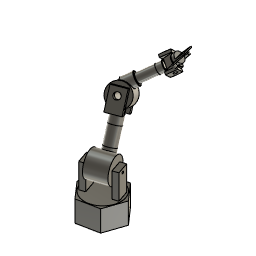
Robotic ARM v11 (Autodesk Fusion 360 design; units mm, degrees)
Autodesk Fusion 360 part; units mm, degrees
(part 1 of 2)
sketch "Sketch7" plane through (0, 0, 0) normal (0, 0, 1) x (1, 0, 0)
  line L0 (526.8037, -602.0614) -> (784.8023, 155.1947)
  line L1 (784.8023, 155.1947) -> (257.9986, 757.2561)
  line L2 (257.9986, 757.2561) -> (-526.8037, 602.0614)
  line L3 (-526.8037, 602.0614) -> (-784.8023, -155.1947)
  line L4 (-784.8023, -155.1947) -> (-257.9986, -757.2561)
  line L5 (-257.9986, -757.2561) -> (526.8037, -602.0614)
  circle A0 centre (0, 0) radius 667.5
  dimension "d16" = 800
  dimension "d17" = 1335
  constraint coincident A0.centre origin
  measures "d16" distance of L0.start A0.centre
  measures "d17" diameter of A0
extrude "Extrude5" add sketch "Sketch7" along normal blind 770 makes body 1
sketch "Sketch8" plane through (0, 0, 0) normal (0, 0, 1) x (1, 0, 0)
  circle A0 centre (0, 0) radius 630
  dimension "d20" = 1260
  constraint coincident A0.centre origin
  measures "d20" diameter of A0
extrude "Extrude6" add sketch "Sketch8" along normal blind 65 from surface at 770 separate body makes body 2
sketch "Sketch9" plane through (0, 0, 835) normal (0, 0, 1) x (-1, 0, 0)
  circle A0 centre (0, 0) radius 630
  line L0 (0, -630) -> (0, 630)
  line L1 (0, -630) -> (0, -480)
  line L2 (0, 630) -> (0, 480)
  line L3 (225, -380) -> (-225, -380)
  line L4 (-225, -380) -> (-225, -580)
  line L5 (-225, -580) -> (225, -580)
  line L6 (225, -580) -> (225, -380)
  line L7 (225, -380) -> (-225, -580) construction
  line L8 (-225, -380) -> (225, -580) construction
  line L9 (-225, 380) -> (225, 380)
  line L10 (225, 380) -> (225, 580)
  line L11 (225, 580) -> (-225, 580)
  line L12 (-225, 580) -> (-225, 380)
  line L13 (-225, 380) -> (225, 580) construction
  line L14 (225, 380) -> (-225, 580) construction
  point P0 (0, -480)
  point P1 (0, 480)
  dimension "d24" = 150
  dimension "d25" = 150
  dimension "d26" = 450
  dimension "d27" = 200
  dimension "d28" = 450
  dimension "d29" = 200
  constraint coincident A0 L0.start
  constraint coincident A0 L0.end
  constraint vertical L0
  constraint parallel L0 L1
  constraint parallel L0 L2
  constraint horizontal L3
  constraint perpendicular L3 L4
  constraint parallel L3 L5
  constraint parallel L4 L6
  constraint coincident L7 P0
  constraint coincident L8 P0
  constraint coincident P0 L1.end
  constraint horizontal L9
  constraint perpendicular L9 L10
  constraint parallel L9 L11
  constraint parallel L10 L12
  constraint coincident L13 P1
  constraint coincident L14 P1
  constraint coincident P1 L2.end
  measures "d24" distance of L0.start P0
  measures "d25" distance of L0.end P1
  measures "d26" distance of L4.end L5.end
  measures "d27" distance of L3.end L4.end
  measures "d28" distance of L10.end L11.end
  measures "d29" distance of L9.end L10.end
extrude "Extrude7" add sketch "Sketch9" along normal blind 900 contours L0 L2 L9 L10 L11 | L0 L2 L9 L11 L12 | L0 L1 L3 L4 L5 | L0 L1 L3 L5 L6 bodies 2
sketch "Sketch10" plane through (0, 580, 0) normal (0, 1, 0) x (-1, 0, 0)
  line L0 (-225, 835) -> (225, 835)
  line L1 (225, 835) -> (225, 1735)
  line L2 (225, 1735) -> (-225, 1735)
  line L3 (-225, 1735) -> (-225, 835)
  line L4 (0, 835) -> (0, 1602)
  circle A0 centre (0, 1602) radius 42
  circle A1 centre (0, 1602) radius 440
  dimension "d32" = 767
  dimension "d33" = 84
  dimension "d34" = 880
  constraint midpoint L0 L4.start
  constraint perpendicular L0 L4
  constraint coincident L4.end A0.centre
  constraint concentric A0 A1
  measures "d32" distance of L4.start L4.end
  measures "d33" diameter of A0
  measures "d34" diameter of A1
extrude "Extrude8" cut sketch "Sketch10" against normal blind 1300 contours A0 bodies 2
sketch "Sketch11" plane through (0, 580, 0) normal (0, 1, 0) x (-1, 0, 0)
  circle A0 centre (0, 1602) radius 42
  line L0 (-225, 835) -> (225, 835)
  line L1 (225, 835) -> (225, 1735)
  line L2 (225, 1735) -> (-225, 1735)
  line L3 (-225, 1735) -> (-225, 835)
  circle A1 centre (0, 1602) radius 440
  dimension "d37" = 880
  constraint concentric A0 A1
  measures "d37" diameter of A1
extrude "Extrude9" add sketch "Sketch11" against normal blind 715 from surface at -225 separate body contours L1 L2 L3 A1 | L1 L2 L3 A1 makes body 3
sketch "Sketch12" plane through (0, 0, 835) normal (0, 0, 1) x (-1, 0, 0)
  line L0 (225, -580) -> (-225, -580)
  line L1 (-225, -580) -> (-225, -380)
  line L2 (-225, -380) -> (225, -380)
  line L3 (225, -380) -> (225, -580)
  line L4 (-225, 580) -> (225, 580)
  line L5 (225, 580) -> (225, 380)
  line L6 (225, 380) -> (-225, 380)
  line L7 (-225, 380) -> (-225, 580)
  circle A0 centre (0, 0) radius 630
  circle A1 centre (200, 0) radius 205
  dimension "d44" = 410
  measures "d44" diameter of A1
sketch "Sketch13" plane through (0, 0, 770) normal (0, 0, -1) x (1, 0, 0)
  circle A0 centre (0, 0) radius 630
  circle A1 centre (0, 0) radius 667
  dimension "d41" = 1334
  constraint concentric A0 A1
  measures "d41" diameter of A1
extrude "Extrude10" add sketch "Sketch13" against normal blind 65 bodies 2
sketch "Sketch14" plane through (0, 0, 0) normal (0, 1, 0) x (1, 0, 0)
sketch "Sketch15" plane through (0, 0, 835) normal (0, 0, 1) x (-1, 0, 0)
copy_body "Body->Comp2" bodies 3 removing the originals makes body 4 in component "old_component (1)"
copy_body "Body->Comp3" bodies 2 removing the originals makes body 5 in component "old_component (2)"
copy_body "Body->Comp4" bodies 1 removing the originals makes body 6 in component "old_component"
extrude "Extrude1" add 1 faces at (176.6231, 355, 1351.5163) along direction (0, 1, 0) blind 20 on bodies 4 bodies 4 in component "old_component (1)"
sketch "Sketch16" plane through (0, 0, 770) normal (0, 0, 1) x (-1, 0, 0)
  circle A0 centre (0, 0) radius 667
  line L0 (225, -580) -> (-225, -580)
  line L1 (-225, -580) -> (-225, -380)
  line L2 (-225, -380) -> (225, -380)
  line L3 (225, -380) -> (225, -580)
  line L4 (-225, 580) -> (225, 580)
  line L5 (225, 580) -> (225, 380)
  line L6 (225, 380) -> (-225, 380)
  line L7 (-225, 380) -> (-225, 580)
  circle A1 centre (200, 0) radius 205
  dimension "d60" = 410
  measures "d60" diameter of A1
extrude "Extrude2" add sketch "Sketch16" along normal blind 400 and the other way blind 0 from surface at 900 contours A1 sketch seen with x (1, 0, 0) y (0, 1, 0) z (0, 0, 1) at (0, 7.5, 65) bodies 4 in component "old_component (1)"
sketch "Sketch17" plane through (0, 0, 1880.3087) normal (0, 0, 1) x (-1, 0, 0)
  circle A0 centre (137.9029, 21.8013) radius 205
  circle A1 centre (137.9029, 21.8013) radius 204
  dimension "d66" = 408
  constraint concentric A0 A1
  measures "d66" diameter of A1
extrude "Extrude3" cut sketch "Sketch17" against normal blind 300 contours A1 sketch seen with x (1, 0, 0) y (0, 1, 0) z (0, 0, 1) at (-62.0971, 29.3013, 254.6913) bodies 4 in component "old_component (1)"
sketch "Sketch18" plane through (0, 0, 1633.8201) normal (0, 0, 1) x (-1, 0, 0)
  circle A0 centre (38.5203, 22.1078) radius 204
extrude "Extrude4" add sketch "Sketch18" along normal blind 1200 sketch seen with x (1, 0, 0) y (0, 1, 0) z (0, 0, 1) at (-161.4797, 29.6078, 201.1799) bodies 4 in component "old_component (1)"
sketch "Sketch19" plane through (0, 0, 2833.8201) normal (0, 0, 1) x (-1, 0, 0)
  circle A0 centre (38.5203, 22.1078) radius 204
  circle A1 centre (38.5203, 22.1078) radius 205
  dimension "d71" = 410
  constraint concentric A0 A1
  measures "d71" diameter of A1
extrude "Extrude12" add sketch "Sketch19" against normal blind 300 separate body contours A0 makes body 7
sketch "Sketch20" plane through (0, 0, 2833.8201) normal (0, 0, 1) x (-1, 0, 0)
  circle A0 centre (38.5203, 22.1078) radius 204
  line L0 (-165.4797, 22.1078) -> (-415.4797, 22.1078)
  line L1 (-415.4797, 22.1078) -> (-415.4797, -227.8922)
  line L2 (-415.4797, 22.1078) -> (-415.4797, 272.1078)
  line L3 (242.5203, 22.1078) -> (492.5203, 22.1078)
  line L4 (492.5203, 22.1078) -> (492.5203, 272.1078)
  line L5 (492.5203, 22.1078) -> (492.5203, -227.8922)
  line L6 (38.5203, 22.1078) -> (-261.4797, 22.1078)
  line L7 (38.5203, 22.1078) -> (338.5203, 22.1078)
  line L8 (338.5203, 22.1078) -> (338.5203, -227.8922)
  line L9 (338.5203, -227.8922) -> (492.5203, -227.8922)
  line L10 (492.5203, 272.1078) -> (338.5203, 272.1078)
  line L11 (338.5203, 272.1078) -> (338.5203, 22.1078)
  line L12 (-261.4797, 22.1078) -> (-261.4797, 272.1078)
  line L13 (-261.4797, 272.1078) -> (-415.4797, 272.1078)
  line L14 (-261.4797, 22.1078) -> (-261.4797, -227.8922)
  line L15 (-261.4797, -227.8922) -> (-415.4797, -227.8922)
  line L16 (-261.4797, 22.1078) -> (-261.4797, 147.1078)
  line L17 (338.5203, 147.1078) -> (338.5203, -102.8922)
  line L18 (-261.4797, -102.8922) -> (338.5203, -102.8922)
  line L19 (338.5203, 147.1078) -> (-261.4797, 147.1078)
  point P0 (-165.4797, 22.1078)
  dimension "d74" = 250
  dimension "d76" = 250
  dimension "d77" = 250
  dimension "d80" = 250
  dimension "d81" = 250
  dimension "d82" = 250
  dimension "d83" = 300
  dimension "d84" = 300
  constraint coincident P0 L0.start
  constraint horizontal L0
  constraint perpendicular L0 L1
  constraint perpendicular L0 L2
  constraint coincident A0 L3.start
  constraint parallel L0 L3
  constraint perpendicular L3 L4
  constraint perpendicular L3 L5
  constraint coincident A0.centre L6.start
  constraint coincident L0 L6.end
  constraint parallel L3 L7
  constraint perpendicular L7 L8
  constraint perpendicular L5 L9
  constraint perpendicular L8 L10
  constraint perpendicular L7 L11
  constraint perpendicular L6 L12
  constraint perpendicular L2 L13
  constraint perpendicular L0 L14
  constraint perpendicular L1 L15
  constraint midpoint L12 L16.end
  constraint midpoint L11 L17.start
  constraint midpoint L8 L17.end
  constraint midpoint L14 L18.start
  constraint perpendicular L8 L18
  measures "d74" distance of P0 L0.end
  measures "d76" distance of L0.end L1.end
  measures "d77" distance of L0.end L2.end
  measures "d80" distance of L3.start L3.end
  measures "d81" distance of L3.end L4.end
  measures "d82" distance of L3.end L5.end
  measures "d83" distance of A0.centre L6.end
  measures "d84" distance of A0.centre L7.end
extrude "Extrude13" add sketch "Sketch20" along normal blind 750 contours A0 L6 L7 L19 | A0 L3 L7 L8 L17 L18 | A0 L3 L7 L11 L17 L19 | A0 L6 L7 L18 | L3 L4 L10 L11 L17 | L3 L5 L8 L9 L17 | A0 L0 L6 L12 L16 L19 | A0 L0 L6 L14 L18 | L0 L2 L12 L13 L16 | L0 L1 L14 L15 bodies 7
sketch "Sketch21" plane through (0, 0, 3583.8201) normal (0, 0, 1) x (-1, 0, 0)
  line L0 (492.5203, -227.8922) -> (492.5203, 272.1078)
  line L1 (492.5203, 272.1078) -> (338.5203, 272.1078)
  line L2 (338.5203, 272.1078) -> (338.5203, 147.1078)
  line L3 (338.5203, 147.1078) -> (-261.4797, 147.1078)
  line L4 (-261.4797, 147.1078) -> (-261.4797, 272.1078)
  line L5 (-261.4797, 272.1078) -> (-415.4797, 272.1078)
  line L6 (-415.4797, 272.1078) -> (-415.4797, -227.8922)
  line L7 (-415.4797, -227.8922) -> (-261.4797, -227.8922)
  line L8 (-261.4797, -227.8922) -> (-261.4797, -102.8922)
  line L9 (-261.4797, -102.8922) -> (338.5203, -102.8922)
  line L10 (338.5203, -102.8922) -> (338.5203, -227.8922)
  line L11 (338.5203, -227.8922) -> (492.5203, -227.8922)
  line L12 (-261.4797, 147.1078) -> (-261.4797, -102.8922)
  line L13 (338.5203, -102.8922) -> (338.5203, 147.1078)
  line L14 (-261.4797, 147.1078) -> (-261.4797, -102.8922)
  line L15 (338.5203, -102.8922) -> (-261.4797, -102.8922)
  line L16 (-261.4797, 147.1078) -> (338.5203, 147.1078)
  constraint coincident L3.end L4.start
  constraint coincident L8.end L9.start
  constraint coincident L9.end L10.start
  constraint coincident L2.end L3.start
extrude "Extrude14" cut sketch "Sketch21" against normal blind 600 contours L3 L9 L12 L13 L14 L15 L16 bodies 7
sketch "Sketch22" plane through (-492.5203, 0, 0) normal (-1, 0, 0) x (0, -1, 0)
  line L0 (-227.8922, 2833.8201) -> (272.1078, 2833.8201)
  line L1 (272.1078, 2833.8201) -> (272.1078, 3583.8201)
  line L2 (272.1078, 3583.8201) -> (-227.8922, 3583.8201)
  line L3 (-227.8922, 3583.8201) -> (-227.8922, 2833.8201)
  line L4 (22.1078, 2833.8201) -> (22.1078, 3333.8201)
  circle A0 centre (22.1078, 3333.8201) radius 112
  dimension "d89" = 500
  dimension "d90" = 224
  constraint midpoint L0 L4.start
  constraint perpendicular L0 L4
  constraint coincident L4.end A0.centre
  measures "d89" distance of L4.start L4.end
  measures "d90" diameter of A0
extrude "Extrude15" cut sketch "Sketch22" against normal blind 2400 contours A0 bodies 7
sketch "Sketch23" plane through (415.4797, 0, 0) normal (1, 0, 0) x (0, 1, 0)
  circle A0 centre (-22.1078, 3333.8201) radius 112
  line L0 (-272.1078, 2833.8201) -> (227.8922, 2833.8201)
  line L1 (227.8922, 2833.8201) -> (227.8922, 3583.8201)
  line L2 (227.8922, 3583.8201) -> (-272.1078, 3583.8201)
  line L3 (-272.1078, 3583.8201) -> (-272.1078, 2833.8201)
  circle A1 centre (-22.1078, 3333.8201) radius 390
  dimension "d97" = 780
  constraint concentric A0 A1
  measures "d97" diameter of A1
extrude "Extrude16" add sketch "Sketch23" against normal blind 600 from surface at -150 separate body contours L1 L2 L3 A1 | L1 L2 L3 A1 makes body 8
sketch "Sketch24" plane through (0, 0, 3583.8201) normal (0, 0, 1) x (-1, 0, 0)
  line L0 (338.5203, 272.1078) -> (338.5203, -227.8922)
  line L1 (338.5203, -227.8922) -> (492.5203, -227.8922)
  line L2 (492.5203, -227.8922) -> (492.5203, 272.1078)
  line L3 (492.5203, 272.1078) -> (338.5203, 272.1078)
  circle A0 centre (33.0014, 228.1503) radius 222.5
  dimension "d101" = 445
  measures "d101" diameter of A0
extrude "Extrude17" add sketch "Sketch24" along normal blind 200 and the other way blind 100 contours A0 bodies 8
extrude "Extrude18" add 1 faces at (-79.2435, -170.1644, 3783.8201) along direction (0, 0, 1) blind 0 and the other way blind 300 separate body on bodies 8 makes body 9
extrude "Extrude19" add 1 faces at (-79.2435, -170.1644, 3783.8201) along direction (0, 0, 1) blind 100 on bodies 8 bodies 8 9
sketch "Sketch25" plane through (0, 0, 3883.8201) normal (0, 0, 1) x (-1, 0, 0)
  circle A0 centre (33.0014, 228.1503) radius 222.5
  circle A1 centre (33.0014, 228.1503) radius 200
  dimension "d112" = 400
  constraint concentric A0 A1
  measures "d112" diameter of A1
extrude "Extrude20" add sketch "Sketch25" along normal blind 15 contours A1 bodies 8
sketch "Sketch26" plane through (0, 0, 3898.8201) normal (0, 0, 1) x (-1, 0, 0)
  circle A0 centre (33.0014, 228.1503) radius 200
  circle A1 centre (33.0014, 228.1503) radius 155
  dimension "d115" = 310
  constraint concentric A0 A1
  measures "d115" diameter of A1
extrude "Extrude21" add sketch "Sketch26" along normal blind 900 separate body contours A1 makes body 10
sketch "Sketch27" plane through (0, 0, 4798.8201) normal (0, 0, 1) x (-1, 0, 0)
  circle A0 centre (33.0014, 228.1503) radius 155
  circle A1 centre (33.0014, 228.1503) radius 162.5
  dimension "d118" = 325
  constraint concentric A0 A1
  measures "d118" diameter of A1
extrude "Extrude22" add sketch "Sketch27" along normal blind 200 separate body makes body 11
sketch "Sketch28" plane through (0, 0, 4998.8201) normal (0, 0, 1) x (-1, 0, 0)
  circle A0 centre (33.0014, 228.1503) radius 155
  circle A1 centre (33.0014, 228.1503) radius 162.5
  circle A2 centre (33.0014, 228.1503) radius 155
  constraint concentric A0 A2
extrude "Extrude23" add sketch "Sketch28" against normal blind 1 contours A0 A2 bodies 11
sketch "Sketch29" plane through (0, 0, 4998.8201) normal (0, 0, 1) x (-1, 0, 0)
  circle A0 centre (33.0014, 228.1503) radius 162.5
  line L0 (33.0014, 228.1503) -> (-171.9986, 228.1503)
  line L1 (-171.9986, 228.1503) -> (238.0014, 228.1503)
  line L2 (-129.4986, 228.1503) -> (-126.7294, 258.0222)
  line L3 (-129.4986, 228.1503) -> (-126.7294, 198.2784)
  line L4 (-126.7294, 198.2784) -> (-171.9986, 198.2784)
  line L5 (-126.7294, 258.0222) -> (-171.9986, 258.0222)
  line L6 (-171.9986, 258.0222) -> (-171.9986, 228.1503)
  line L7 (-171.9986, 198.2784) -> (-171.9986, 228.1503)
  line L8 (195.5014, 228.1503) -> (192.7321, 258.0222)
  line L9 (195.5014, 228.1503) -> (192.7203, 198.2155)
  line L10 (238.0014, 228.1503) -> (238.0014, 198.2155)
  line L11 (238.0014, 198.2155) -> (192.7203, 198.2155)
  line L12 (238.0014, 258.0222) -> (192.7321, 258.0222)
  line L13 (238.0014, 258.0222) -> (238.0014, 228.1503)
  point P0 (-129.4986, 228.1503)
  dimension "d123" = 205
  dimension "d124" = 410
  dimension "d126" = 30
  dimension "d127" = 30
  dimension "d128" = 30
  constraint coincident A0.centre L0.start
  constraint horizontal L0
  constraint parallel L0 L1
  constraint coincident P0 L2.start
  constraint coincident A0 L2.end
  constraint coincident A0 L3.end
  constraint parallel L1 L4
  constraint parallel L0 L5
  constraint perpendicular L5 L6
  constraint perpendicular L1 L7
  constraint coincident L1 L8.start
  constraint coincident A0 L8.start
  constraint coincident A0 L8.end
  constraint coincident A0 L9.end
  constraint perpendicular L1 L10
  constraint perpendicular L10 L11
  constraint parallel L1 L12
  constraint perpendicular L1 L13
  measures "d123" distance of A0.centre L0.end
  measures "d124" distance of L0.end L1.end
  measures "d126" distance of P0 L2.end
  measures "d127" distance of P0 L3.end
  measures "d128" distance of L8.start L8.end
extrude "Extrude24" add sketch "Sketch29" along normal blind 10 contours A0 L1 L10 L11 | A0 L1 L12 L13 | A0 L0 L1 L5 L6 | A0 L0 L1 L4 L7 bodies 11
sketch "Sketch30" plane through (0, 0, 5008.8201) normal (0, 0, 1) x (-1, 0, 0)
  line L0 (-126.7294, 258.0222) -> (-171.9986, 258.0222)
  line L1 (-171.9986, 258.0222) -> (-171.9986, 198.2784)
  line L2 (-171.9986, 198.2784) -> (-126.7294, 198.2784)
  arc A0 (-126.7294, 258.0222) -> (-126.7294, 198.2784) centre (33.0014, 228.1503) ccw
  line L3 (-171.9986, 198.2784) -> (-171.9986, 48.2784)
  line L4 (-171.9986, 258.0222) -> (-171.9986, 408.0222)
  line L5 (-171.9986, 408.0222) -> (-261.9986, 408.0222)
  line L6 (-261.9986, 408.0222) -> (-261.9986, 48.2784)
  line L7 (-261.9986, 48.2784) -> (-171.9986, 48.2784)
  line L8 (-171.9986, 198.2784) -> (-171.9986, 258.0222)
  line L9 (238.0014, 258.0222) -> (238.0014, 408.0222)
  line L10 (238.0014, 198.2155) -> (238.0014, 258.0222)
  line L11 (238.0014, 258.0222) -> (238.0014, 198.2832)
  line L12 (238.0014, 198.2832) -> (238.0014, 48.2832)
  line L13 (238.0014, 48.2832) -> (328.0014, 48.2832)
  line L14 (328.0014, 48.2832) -> (328.0014, 408.0222)
  line L15 (328.0014, 408.0222) -> (238.0014, 408.0222)
  point P0 (238.0014, 258.0222)
  dimension "d131" = 150
  dimension "d132" = 150
  dimension "d133" = 90
  dimension "d134" = 150
  dimension "d135" = 150
  dimension "d136" = 90
  constraint coincident L1.end L2.start
  constraint perpendicular L2 L3
  constraint coincident L0.end L1.start
  constraint perpendicular L0 L4
  constraint perpendicular L4 L5
  constraint perpendicular L0 L6
  constraint perpendicular L3 L7
  constraint coincident P0 L9.start
  constraint vertical L9
  constraint coincident L10 L11.end
  constraint parallel L9 L11
  constraint parallel L11 L12
  constraint perpendicular L12 L13
  constraint perpendicular L13 L14
  constraint perpendicular L9 L15
  measures "d131" distance of L1.end L3.end
  measures "d132" distance of L0.end L4.end
  measures "d133" distance of L4.end L5.end
  measures "d134" distance of P0 L9.end
  measures "d135" distance of L11.end L12.end
  measures "d136" distance of L12.end L13.end
extrude "Extrude25" add sketch "Sketch30" along normal blind -10 and the other way blind -400 contours L1 L3 L4 L5 L6 L7 L8 | L9 L10 L11 L12 L13 L14 L15 bodies 11 10 8 7
sketch "Sketch31" plane through (-328.0014, 0, 0) normal (-1, 0, 0) x (0, -1, 0)
  line L0 (48.2832, 5408.8201) -> (48.2832, 4998.8201)
  line L1 (48.2832, 4998.8201) -> (408.0222, 4998.8201)
  line L2 (408.0222, 4998.8201) -> (408.0222, 5408.8201)
  line L3 (408.0222, 5408.8201) -> (48.2832, 5408.8201)
  line L4 (408.0222, 4998.8201) -> (48.2832, 4998.8201)
  line L5 (228.1527, 4998.8201) -> (228.1527, 5148.8201)
  circle A0 centre (228.1527, 5218.8201) radius 70
  dimension "d141" = 150
  dimension "d142" = 140
  constraint coincident L1.end L2.start
  constraint coincident L0.end L1.start
  constraint midpoint L4 L5.start
  constraint perpendicular L4 L5
  constraint coincident L5.end A0
  measures "d141" distance of L5.start L5.end
  measures "d142" diameter of A0
extrude "Extrude26" cut sketch "Sketch31" against normal blind 1400 contours A0 bodies 11
sketch "Sketch32" plane through (261.9986, 0, 0) normal (1, 0, 0) x (0, 1, 0)
  circle A0 centre (-228.1527, 5218.8201) radius 70
  line L0 (-408.0222, 5408.8201) -> (-408.0222, 4998.8201)
  line L1 (-408.0222, 4998.8201) -> (-48.2784, 4998.8201)
  line L2 (-48.2784, 4998.8201) -> (-48.2784, 5408.8201)
  line L3 (-48.2784, 5408.8201) -> (-408.0222, 5408.8201)
  line L4 (-228.1527, 5218.8201) -> (-228.1527, 5048.8201)
  line L5 (-228.1527, 5218.8201) -> (-228.1527, 5388.8201)
  line L6 (-228.1527, 5388.8201) -> (-398.1527, 5388.8201)
  line L7 (-228.1527, 5388.8201) -> (-58.1527, 5388.8201)
  line L8 (-58.1527, 5388.8201) -> (-58.1527, 5048.8201)
  line L9 (-58.1527, 5048.8201) -> (-228.1527, 5048.8201)
  line L10 (-398.1527, 5388.8201) -> (-398.1527, 5048.8201)
  line L11 (-398.1527, 5048.8201) -> (-228.1527, 5048.8201)
  dimension "d145" = 170
  dimension "d146" = 170
  dimension "d147" = 170
  dimension "d148" = 170
  constraint coincident A0.centre L4.start
  constraint vertical L4
  constraint parallel L4 L5
  constraint perpendicular L5 L6
  constraint perpendicular L5 L7
  constraint perpendicular L7 L8
  constraint perpendicular L4 L9
  constraint perpendicular L6 L10
  constraint perpendicular L4 L11
  measures "d145" distance of A0.centre L4.end
  measures "d146" distance of A0.centre L5.end
  measures "d147" distance of L5.end L6.end
  measures "d148" distance of L5.end L7.end
extrude "Extrude27" add sketch "Sketch32" against normal blind 400 from surface at -95 separate body contours A0 L4 L5 | A0 L4 L5 L7 L8 L9 | A0 L4 L5 | A0 L4 L5 L6 L10 L11 makes body 12
extrude "Extrude28" cut 1 faces at (231.9986, -168.193, 5408.8201) along direction (0, 0, -1) blind 50 on bodies 11 bodies 11
extrude "Extrude29" cut 1 faces at (-298.0014, -288.1092, 5408.8201) along direction (0, 0, -1) blind 50 on bodies 11 bodies 11
sketch "Sketch33" plane through (-233.0014, 0, 0) normal (-1, 0, 0) x (0, -1, 0)
  line L0 (398.1527, 5388.8201) -> (58.1527, 5388.8201)
  line L1 (58.1527, 5388.8201) -> (58.1527, 5048.8201)
  line L2 (58.1527, 5048.8201) -> (398.1527, 5048.8201)
  line L3 (398.1527, 5048.8201) -> (398.1527, 5388.8201)
  circle A0 centre (228.1527, 5218.8201) radius 30
  dimension "d156" = 60
  measures "d156" diameter of A0
extrude "Extrude30" cut sketch "Sketch33" against normal blind 900 contours A0 bodies 12
sketch "Sketch34" plane through (0, 0, 5388.8201) normal (0, 0, 1) x (-1, 0, 0)
  line L0 (-166.9986, 398.1527) -> (-166.9986, 58.1527)
  line L1 (-166.9986, 58.1527) -> (233.0014, 58.1527)
  line L2 (233.0014, 58.1527) -> (233.0014, 398.1527)
  line L3 (233.0014, 398.1527) -> (-166.9986, 398.1527)
  line L4 (-166.9986, 228.1527) -> (233.0014, 228.1527)
  line L5 (33.0014, 228.1527) -> (33.0014, 58.1527)
  circle A0 centre (33.0014, 228.1527) radius 180
  dimension "d159" = 360
  constraint midpoint L0 L4.start
  constraint midpoint L2 L4.end
  constraint midpoint L4 L5.start
  constraint midpoint L1 L5.end
  constraint coincident L5.start A0.centre
  measures "d159" diameter of A0
extrude "Extrude31" add sketch "Sketch34" along normal blind 30 contours L3 A0 | L3 L4 A0 | L1 L4 L5 A0 | L1 A0 | L1 L4 L5 A0 bodies 12
extrude "Extrude32" add 1 faces at (-52.7216, -58.1527, 5162.1535) along direction (0, 1, 0) blind 10 on bodies 12 bodies 12
extrude "Extrude33" add 1 faces at (-52.7216, -398.1527, 5162.1535) along direction (0, -1, 0) blind 10 on bodies 12 bodies 12
sketch "Sketch35" plane through (0, 0, 5418.8201) normal (0, 0, 1) x (-1, 0, 0)
  circle A0 centre (33.0014, 228.1527) radius 180
  circle A1 centre (33.0014, 228.1527) radius 180
  dimension "d166" = 360
  constraint concentric A0 A1
  measures "d166" diameter of A1
extrude "Extrude34" add sketch "Sketch35" along normal blind 90 separate body makes body 13
sketch "Sketch36" plane through (0, 0, 5508.8201) normal (0, 0, 1) x (-1, 0, 0)
  circle A0 centre (33.0014, 228.1527) radius 180
  circle A1 centre (33.0014, 228.1527) radius 180
  dimension "d169" = 360
  constraint concentric A0 A1
  measures "d169" diameter of A1
extrude "Extrude35" add sketch "Sketch36" along normal blind 30 bodies 13
sketch "Sketch37" plane through (0, 0, 5538.8201) normal (0, 0, 1) x (-1, 0, 0)
  circle A0 centre (33.0014, 228.1527) radius 180
  line L0 (33.0014, 228.1527) -> (213.0014, 228.1527)
  line L1 (33.0014, 228.1527) -> (-146.9986, 228.1527)
  line L2 (-146.9986, 228.1527) -> (-146.9986, 188.1527)
  line L3 (213.0014, 228.1527) -> (213.0014, 188.1527)
  line L4 (213.0014, 188.1527) -> (-146.9986, 188.1527)
  dimension "d172" = 180
  dimension "d173" = 40
  dimension "d174" = 40
  constraint coincident A0.centre L0.start
  constraint coincident A0 L0.end
  constraint horizontal L0
  constraint parallel L0 L1
  constraint perpendicular L1 L2
  constraint tangent A0 L3
  measures "d172" distance of A0.centre L1.end
  measures "d173" distance of L1.end L2.end
  measures "d174" distance of L0.end L3.end
extrude "Extrude36" add sketch "Sketch37" along normal blind 390 contours A0 L0 L1 L4 bodies 13
sketch "Sketch38" plane through (0, -228.1527, 0) normal (0, -1, 0) x (1, 0, 0)
  line L0 (-213.0014, 5538.8201) -> (146.9986, 5538.8201)
  line L1 (146.9986, 5538.8201) -> (146.9986, 5928.8201)
  line L2 (146.9986, 5928.8201) -> (-213.0014, 5928.8201)
  line L3 (-213.0014, 5928.8201) -> (-213.0014, 5538.8201)
  line L4 (-213.0014, 5538.8201) -> (-100.5104, 5538.8201)
  line L5 (-100.5104, 5538.8201) -> (-100.5104, 5639.8161)
  circle A0 centre (-100.5104, 5639.8161) radius 20
  dimension "d177" = 112.491
  dimension "d178" = 100.996
  dimension "d179" = 40
  constraint coincident L0.start L3.end
  constraint coincident L0 L4.end
  constraint perpendicular L4 L5
  constraint coincident L5.end A0.centre
  measures "d177" distance of L0.start L4.end
  measures "d178" distance of L4.end L5.end
  measures "d179" diameter of A0
extrude "Extrude37" cut sketch "Sketch38" against normal blind 1175 contours A0 bodies 13
sketch "Sketch39" plane through (0, -228.1527, 0) normal (0, -1, 0) x (1, 0, 0)
  circle A0 centre (-100.5104, 5639.8161) radius 20
  line L0 (-213.0014, 5538.8201) -> (146.9986, 5538.8201)
  line L1 (146.9986, 5538.8201) -> (146.9986, 5928.8201)
  line L2 (146.9986, 5928.8201) -> (-213.0014, 5928.8201)
  line L3 (-213.0014, 5928.8201) -> (-213.0014, 5538.8201)
  line L4 (146.9986, 5538.8201) -> (34.5076, 5538.8201)
  line L5 (34.5076, 5538.8201) -> (34.5076, 5639.8161)
  circle A1 centre (34.5076, 5639.8161) radius 20
  dimension "d182" = 112.491
  dimension "d183" = 40
  constraint coincident L0.end L1.start
  constraint perpendicular L1 L4
  constraint perpendicular L4 L5
  constraint coincident L5.end A1.centre
  measures "d182" distance of L0.end L4.end
  measures "d183" diameter of A1
extrude "Extrude38" cut sketch "Sketch39" against normal blind 250 contours A1 bodies 13
sketch "Sketch40" plane through (0, -228.1527, 0) normal (0, -1, 0) x (1, 0, 0)
  circle A0 centre (34.5076, 5639.8161) radius 20
  circle A1 centre (-100.5104, 5639.8161) radius 20
  line L0 (-213.0014, 5538.8201) -> (146.9986, 5538.8201)
  line L1 (146.9986, 5538.8201) -> (146.9986, 5928.8201)
  line L2 (146.9986, 5928.8201) -> (-213.0014, 5928.8201)
  line L3 (-213.0014, 5928.8201) -> (-213.0014, 5538.8201)
  line L4 (-213.0014, 5928.8201) -> (-85.0624, 5928.8201)
  line L5 (-85.0624, 5928.8201) -> (-85.0624, 5833.2951)
  line L6 (146.9986, 5928.8201) -> (19.0596, 5928.8201)
  line L7 (19.0596, 5928.8201) -> (19.0596, 5833.2951)
  circle A2 centre (19.0596, 5833.2951) radius 20
  circle A3 centre (-85.0624, 5833.2951) radius 20
  dimension "d186" = 127.939
  dimension "d187" = 95.525
  dimension "d188" = 127.939
  dimension "d189" = 95.525
  dimension "d190" = 40
  dimension "d191" = 40
  constraint coincident L2.end L3.start
  constraint perpendicular L3 L4
  constraint perpendicular L4 L5
  constraint coincident L1.end L2.start
  constraint perpendicular L1 L6
  constraint perpendicular L2 L7
  constraint coincident L7.end A2.centre
  constraint coincident L5.end A3.centre
  measures "d186" distance of L2.end L4.end
  measures "d187" distance of L4.end L5.end
  measures "d188" distance of L1.end L6.end
  measures "d189" distance of L6.end L7.end
  measures "d190" diameter of A2
  measures "d191" diameter of A3
extrude "Extrude39" cut sketch "Sketch40" against normal blind 150 contours A2 | A3 bodies 13
sketch "Sketch41" plane through (0, -228.1527, 0) normal (0, -1, 0) x (1, 0, 0)
  circle A0 centre (19.0596, 5833.2951) radius 20
  circle A1 centre (-85.0624, 5833.2951) radius 20
  circle A2 centre (34.5076, 5639.8161) radius 20
  circle A3 centre (-100.5104, 5639.8161) radius 20
  line L0 (-213.0014, 5538.8201) -> (146.9986, 5538.8201)
  line L1 (146.9986, 5538.8201) -> (146.9986, 5928.8201)
  line L2 (146.9986, 5928.8201) -> (-213.0014, 5928.8201)
  line L3 (-213.0014, 5928.8201) -> (-213.0014, 5538.8201)
  line L4 (19.0596, 5833.2951) -> (342.5354, 6163.1548)
  circle A4 centre (342.5354, 6163.1548) radius 20
  circle A5 centre (19.0596, 5833.2951) radius 20
  line L5 (342.5354, 6163.1548) -> (356.8151, 6149.1516)
  line L6 (356.8151, 6149.1516) -> (33.3393, 5819.2919)
  line L7 (19.0596, 5833.2951) -> (4.78, 5847.2984)
  line L8 (4.78, 5847.2984) -> (328.2558, 6177.1581)
  circle A6 centre (342.5354, 6163.1548) radius 32.5
  circle A7 centre (19.0596, 5833.2951) radius 32.5
  circle A8 centre (-85.0624, 5833.2951) radius 32.5
  circle A9 centre (-85.0624, 5833.2951) radius 20
  line L9 (-85.0624, 5833.2951) -> (-299.774, 6242.3708)
  circle A10 centre (-299.774, 6242.3708) radius 20
  circle A11 centre (-299.774, 6242.3708) radius 32.5
  line L10 (-85.0624, 5833.2951) -> (-102.7713, 5824.0003)
  line L11 (-85.0624, 5833.2951) -> (-67.3535, 5842.59)
  line L12 (-102.7713, 5824.0003) -> (-317.4829, 6233.076)
  line L13 (-299.774, 6242.3708) -> (-282.0651, 6251.6657)
  line L14 (-282.0651, 6251.6657) -> (-67.3535, 5842.59)
  dimension "d194" = 462
  dimension "d195" = 40
  dimension "d196" = 40
  dimension "d197" = 65
  dimension "d198" = 65
  dimension "d199" = 65
  dimension "d200" = 40
  dimension "d201" = 462
  dimension "d202" = 40
  dimension "d203" = 65
  constraint coincident A0.centre L4.start
  constraint coincident L4.end A4.centre
  constraint coincident A4 L5.end
  constraint perpendicular L4 L5
  constraint coincident A5 L6.end
  constraint tangent A5 L6
  constraint coincident A5 L7.end
  constraint perpendicular L4 L7
  constraint coincident A4 L8.end
  constraint tangent A4 L8
  constraint concentric A4 A6
  constraint concentric A1 A8
  constraint concentric A8 A9
  constraint coincident A1.centre A8.centre
  constraint coincident L9.end A10.centre
  constraint coincident A9 L10.end
  constraint perpendicular L9 L10
  constraint coincident A9 L11.end
  constraint perpendicular L9 L11
  constraint coincident A10 L12.end
  constraint tangent A10 L12
  constraint coincident A10 L13.end
  constraint perpendicular L9 L13
  measures "d194" distance of A0.centre L4.end
  measures "d195" diameter of A4
  measures "d196" diameter of A5
  measures "d197" diameter of A6
  measures "d198" diameter of A7
  measures "d199" diameter of A8
  measures "d200" diameter of A9
  measures "d201" distance of A1.centre L9.end
  measures "d202" diameter of A10
  measures "d203" diameter of A11
extrude "Extrude40" add sketch "Sketch41" along normal blind 40 separate body contours A0 L4 A5 L8 A7 | A0 A5 L6 L8 A7 | A0 L4 A5 L6 A7 | L2 L4 L8 A7 | L2 L4 L6 A7 | L2 L4 L8 A6 | L2 L4 L6 A6 | L2 A8 L9 L14 | L2 L9 A11 L14 | A4 L6 L8 A6 | L4 A4 L8 A6 | L4 A4 L6 A6 | L2 A8 L9 L12 | L2 L9 A11 L12 | A10 A11 L12 L14 | L9 A10 A11 L14 | A1 A8 A9 L9 L14 | A1 A8 A9 L12 L14 | A1 A8 A9 L9 L12 | L9 A10 A11 L12 makes body 14 at (-154.6984, -228.1527, 5980.3129) makes body 15 at (137.6236, -228.1527, 5944.6774)
sketch "Sketch42" plane through (0, -228.1527, 0) normal (0, -1, 0) x (1, 0, 0)
  circle A0 centre (19.0596, 5833.2951) radius 20
  circle A1 centre (-85.0624, 5833.2951) radius 20
  circle A2 centre (34.5076, 5639.8161) radius 20
  circle A3 centre (-100.5104, 5639.8161) radius 20
  line L0 (-213.0014, 5538.8201) -> (146.9986, 5538.8201)
  line L1 (146.9986, 5538.8201) -> (146.9986, 5928.8201)
  line L2 (146.9986, 5928.8201) -> (-213.0014, 5928.8201)
  line L3 (-213.0014, 5928.8201) -> (-213.0014, 5538.8201)
  circle A4 centre (-100.5104, 5639.8161) radius 20
  line L4 (-100.5104, 5639.8161) -> (-409.6389, 5972.1034)
  circle A5 centre (-409.6389, 5972.1034) radius 20
  circle A6 centre (34.5076, 5639.8161) radius 20
  line L5 (34.5076, 5639.8161) -> (437.9419, 5847.7009)
  circle A7 centre (437.9419, 5847.7009) radius 20
  circle A8 centre (-100.5104, 5639.8161) radius 65
  circle A9 centre (34.5076, 5639.8161) radius 65
  line L6 (34.5076, 5639.8161) -> (4.7342, 5697.5963)
  line L7 (34.5076, 5639.8161) -> (64.2811, 5582.036)
  line L8 (-100.5104, 5639.8161) -> (-148.1008, 5595.5425)
  line L9 (-100.5104, 5639.8161) -> (-52.9199, 5684.0897)
  circle A10 centre (437.9419, 5847.7009) radius 40
  circle A11 centre (-409.6389, 5972.1034) radius 40
  line L10 (64.2811, 5582.036) -> (458.1874, 5813.2028)
  line L11 (4.7342, 5697.5963) -> (421.5984, 5884.2097)
  line L12 (-52.9199, 5684.0897) -> (-381.8915, 6000.9146)
  line L13 (-148.1008, 5595.5425) -> (-440.3761, 5946.5061)
  dimension "d206" = 40
  dimension "d207" = 453.845
  dimension "d208" = 40
  dimension "d209" = 40
  dimension "d210" = 453.845
  dimension "d211" = 40
  dimension "d212" = 130
  dimension "d213" = 130
  dimension "d214" = 80
  dimension "d215" = 80
  constraint concentric A3 A4
  constraint coincident A3.centre A4.centre
  constraint coincident L4.end A5.centre
  constraint concentric A2 A6
  constraint coincident A2.centre A6.centre
  constraint coincident L5.end A7.centre
  constraint concentric A4 A8
  constraint concentric A2 A9
  constraint coincident A9 L6.end
  constraint perpendicular L5 L6
  constraint coincident A9 L7.end
  constraint parallel L6 L7
  constraint coincident A8 L8.end
  constraint perpendicular L4 L8
  constraint coincident A8 L9.end
  constraint perpendicular L4 L9
  constraint concentric A7 A10
  constraint concentric A5 A11
  constraint coincident A10 L10.end
  constraint tangent A10 L10
  constraint coincident A10 L11.end
  constraint tangent A10 L11
  constraint coincident A11 L12.end
  constraint tangent A11 L12
  constraint coincident A11 L13.end
  constraint tangent A11 L13
  measures "d206" diameter of A4
  measures "d207" distance of A3.centre L4.end
  measures "d208" diameter of A5
  measures "d209" diameter of A6
  measures "d210" distance of A2.centre L5.end
  measures "d211" diameter of A7
  measures "d212" diameter of A8
  measures "d213" diameter of A9
  measures "d214" diameter of A10
  measures "d215" diameter of A11
extrude "Extrude41" add sketch "Sketch42" along normal blind 40 separate body contours A2 A6 L5 A9 L7 L10 | A2 A6 L5 A9 L6 L11 | A2 A6 A9 L6 L7 | L1 L5 A9 L11 | L1 L5 A9 L10 | L1 L5 A10 L10 | L1 L5 A10 L11 | A10 | L3 L4 A11 L13 | L3 L4 A8 L13 | L3 L4 A8 L12 | L3 L4 A11 L12 | A3 A4 L4 A8 L8 L13 | A11 | A3 A4 L4 A8 L9 L12 | A3 A4 A8 L8 L9 makes body 16 at (156.5512, -268.1527, 5733.5833) makes body 17 at (-222.9875, -268.1527, 5732.5074)
copy_body "Body->Comp5" bodies 7 removing the originals makes body 18 in component "old_component (3)"
copy_body "Body->Comp6" bodies 8 removing the originals makes body 19 in component "old_component (4)"
copy_body "Body->Comp7" bodies 10 removing the originals makes body 20 in component "old_component (5)"
copy_body "Body->Comp8" bodies 11 removing the originals makes body 21 in component "old_component (6)"
sketch "Sketch43" plane through (0, 0, 3898.8201) normal (0, 0, 1) x (-1, 0, 0)
  circle A0 centre (37.0014, 228.1503) radius 200
  circle A1 centre (37.0014, 228.1503) radius 155
  dimension "d238" = 310
  constraint concentric A0 A1
  measures "d238" diameter of A1
extrude "Extrude1'" cut sketch "Sketch43" against normal blind 101 contours A1 sketch seen with x (1, 0, 0) y (0, 1, 0) z (0, 0, 1) at (4, 0, 0) bodies 19 in component "old_component (4)"
copy_body "Body->Comp9" bodies 12 removing the originals makes body 22 in component "old_component (7)"
copy_body "Body->Comp10" bodies 13 removing the originals makes body 23 in component "old_component (8)"
copy_body "Body->Comp11" bodies 14 removing the originals makes body 24 in component "old_component (9)"
copy_body "Body->Comp12" bodies 15 removing the originals makes body 25 in component "old_component (10)"
copy_body "Body->Comp13" bodies 16 removing the originals makes body 26 in component "old_component (11)"
copy_body "Body->Comp14" bodies 17 removing the originals makes body 27 in component "old_component (12)"
extrude "Extrude1''" cut 1 faces at (-33.0014, -48.1527, 5162.1535) faces seen with x (0.89078, -0.454435, 0) y (0.415957, 0.815355, -0.402711) z (0.183006, 0.358727, 0.915327) at (-863.7789, -1929.2546, 151.0125) along direction (-0.415957, -0.815355, 0.402711) blind 100 on bodies 22 bodies 20 in component "old_component (5)"
extrude "Extrude1'''" cut 1 faces at (-33.0014, -48.1527, 5162.1535) faces seen with x (1, 0, 0) y (0, 0.915327, -0.402711) z (0, 0.402711, 0.915327) at (0, -2120.9942, 350.0125) along direction (0, -0.915327, 0.402711) blind 100 on bodies 22 bodies 21 in component "old_component (6)"
extrude "Extrude1''''" cut 1 faces at (-33.0014, -48.1527, 5162.1535) along direction (0, -1, 0) blind 100 on bodies 22 bodies 22 in component "old_component (7)"
sketch "Sketch44" plane through (280.3092, 299.2761, 207.1799) normal (-0.610143, -0.651427, -0.450964) x (0.729856, -0.683601, 0)
  circle A0 centre (-2437.1103, 2867.216) radius 20
  circle A1 centre (-2426.7372, 2413.4895) radius 20
  line L0 (-2386.7577, 2412.2082) -> (-2372.1273, 2868.7016)
  arc A2 (-2372.1273, 2868.7016) -> (-2502.0934, 2865.7303) centre (-2437.1103, 2867.216) ccw
  line L1 (-2502.0934, 2865.7303) -> (-2466.6163, 2410.3825)
  arc A3 (-2466.6163, 2410.3825) -> (-2386.7577, 2412.2082) centre (-2426.7372, 2413.4895) ccw
  circle A4 centre (-2426.7372, 2413.4895) radius 20
  circle A5 centre (-2642.5776, 2250.3494) radius 20
  circle A6 centre (-2642.5776, 2250.3494) radius 20
  circle A7 centre (-2933.9097, 2397.9351) radius 20
  arc A8 (-2932.0173, 2430.38) -> (-2901.975, 2403.9705) centre (-2933.9097, 2397.9351) ccw
  circle A9 centre (-2921.2628, 2652.8846) radius 20
  circle A10 centre (-2921.2628, 2652.8846) radius 20
  circle A11 centre (-2426.7372, 2413.4895) radius 40
  circle A12 centre (-2642.5776, 2250.3494) radius 40
  circle A13 centre (-2933.9097, 2397.9351) radius 40
  circle A14 centre (-2921.2628, 2652.8846) radius 40
  line L2 (-2426.7372, 2413.4895) -> (-2642.5776, 2250.3494)
  line L3 (-2426.7372, 2413.4895) -> (-2438.7967, 2429.4447)
  line L4 (-2426.7372, 2413.4895) -> (-2414.6776, 2397.5343)
  line L5 (-2438.7967, 2429.4447) -> (-2654.6371, 2266.3046)
  line L6 (-2414.6776, 2397.5343) -> (-2630.5181, 2234.3942)
  line L7 (-2933.9097, 2397.9351) -> (-2921.2628, 2652.8846)
  line L8 (-2921.2628, 2652.8846) -> (-2941.2382, 2653.8755)
  line L9 (-2921.2628, 2652.8846) -> (-2901.2873, 2651.8937)
  line L10 (-2941.2382, 2653.8755) -> (-2953.8852, 2398.926)
  line L11 (-2901.2873, 2651.8937) -> (-2913.9343, 2396.9442)
  line L12 (-2654.6371, 2266.3046) -> (-2618.4586, 2218.439)
  line L13 (-2642.5776, 2250.3494) -> (-2666.6967, 2282.2598)
  line L14 (-2933.9097, 2397.9351) -> (-2893.9097, 2397.9351)
  line L15 (-2933.9097, 2397.9351) -> (-2973.9097, 2397.9351)
  line L16 (-2973.9097, 2397.9351) -> (-2618.4586, 2218.439)
  line L17 (-2796.1842, 2308.1871) -> (-2976.491, 1951.1304)
  line L18 (-2642.5776, 2250.3494) -> (-2796.1842, 2308.1871)
  line L19 (-2976.491, 1951.1304) -> (-2618.4586, 2218.439)
  dimension "d285" = 40
  dimension "d286" = 40
  dimension "d287" = 40
  dimension "d288" = 40
  dimension "d289" = 80
  dimension "d290" = 80
  dimension "d291" = 80
  dimension "d292" = 80
  dimension "d293" = 400
  constraint concentric A1 A4
  constraint concentric A5 A6
  constraint concentric A7 A8
  constraint concentric A9 A10
  constraint concentric A4 A11
  constraint concentric A5 A12
  constraint concentric A8 A13
  constraint concentric A9 A14
  constraint coincident A1.centre A3.centre
  constraint coincident A5.centre A6.centre
  constraint coincident A1 L3.end
  constraint perpendicular L2 L3
  constraint coincident A4 L4.end
  constraint perpendicular L2 L4
  constraint coincident A5 L5.end
  constraint tangent A5 L5
  constraint coincident A6 L6.end
  constraint tangent A6 L6
  constraint coincident A7.centre A8.centre
  constraint coincident A9.centre A10.centre
  constraint coincident A10 L8.end
  constraint perpendicular L7 L8
  constraint coincident A10 L9.end
  constraint perpendicular L7 L9
  constraint coincident A7 L10.end
  constraint tangent A7 L10
  constraint coincident A7 L11.end
  constraint tangent A7 L11
  constraint coincident A12 L12.end
  constraint perpendicular L2 L12
  constraint coincident A12 L13.end
  constraint perpendicular L2 L13
  constraint coincident A13 L14.end
  constraint horizontal L14
  constraint coincident A13 L15.end
  constraint parallel L14 L15
  constraint midpoint L16 L17.start
  constraint perpendicular L16 L17
  measures "d285" diameter of A4
  measures "d286" diameter of A5
  measures "d287" diameter of A7
  measures "d288" diameter of A9
  measures "d289" diameter of A11
  measures "d290" diameter of A12
  measures "d291" diameter of A13
  measures "d292" diameter of A14
  measures "d293" distance of L17.start L17.end
extrude "Extrude42" add sketch "Sketch44" along normal blind 100 separate body contours A1 A3 A4 A11 L5 L6 | A1 A3 A4 A11 L2 L5 | A1 A3 A4 A11 L2 L6 | A3 A11 A12 L2 L5 | A3 A11 A12 L2 L6 | A12 L5 L13 | A5 A6 A12 L2 L5 | A5 A6 A12 L2 L6 | A12 L6 L12 | A5 A6 A12 L13 L18 | A5 A6 L12 L16 | A5 A6 A12 L16 L18 | A12 L16 L17 L19 | A5 A6 A12 L16 makes body 28
sketch "Sketch45" plane through (280.3092, 299.2761, 207.1799) normal (-0.610143, -0.651427, -0.450964) x (0.729856, -0.683601, 0)
  circle A0 centre (-2933.9097, 2397.9351) radius 20
  circle A1 centre (-2628.8802, 2744.9236) radius 20
  arc A2 (-2932.0173, 2430.38) -> (-2901.975, 2403.9705) centre (-2933.9097, 2397.9351) ccw
  line L0 (-2901.975, 2403.9705) -> (-2630.7726, 2712.4787)
  arc A3 (-2630.7726, 2712.4787) -> (-2660.8149, 2738.8882) centre (-2628.8802, 2744.9236) ccw
  line L1 (-2660.8149, 2738.8882) -> (-2932.0173, 2430.38)
  circle A4 centre (-2933.9097, 2397.9351) radius 20
  circle A5 centre (-2933.9097, 2397.9351) radius 40
  arc A6 (-2947.0415, 2683.4698) -> (-2898.9906, 2619.6588) centre (-2921.2628, 2652.8846) ccw
  circle A7 centre (-2921.2628, 2652.8846) radius 20
  circle A8 centre (-2921.2628, 2652.8846) radius 40
  line L2 (-2933.9097, 2397.9351) -> (-2921.2628, 2652.8846)
  line L3 (-2933.9097, 2397.9351) -> (-2973.8606, 2399.9169)
  line L4 (-2933.9097, 2397.9351) -> (-2893.9589, 2395.9533)
  line L5 (-2953.8852, 2398.926) -> (-2941.2382, 2653.8755)
  line L6 (-2913.9343, 2396.9442) -> (-2901.2873, 2651.8937)
  line L7 (-2976.491, 1951.1304) -> (-2973.8606, 2399.9169)
  line L8 (-2976.491, 1951.1304) -> (-2800, 2300)
  line L9 (-2976.491, 1951.1304) -> (-2795.9246, 2308.0559)
  line L10 (-2795.9246, 2308.0559) -> (-2973.8606, 2399.9169)
  point P0 (-2976.491, 1951.1304)
  dimension "d296" = 40
  dimension "d297" = 80
  dimension "d298" = 40
  dimension "d299" = 80
  dimension "d300" = 400
  constraint concentric A0 A4
  constraint concentric A4 A5
  constraint concentric A6 A7
  constraint concentric A6 A8
  constraint coincident A0.centre A2.centre
  constraint coincident A6.centre A7.centre
  constraint coincident A5 L3.end
  constraint perpendicular L2 L3
  constraint coincident A5 L4.end
  constraint parallel L3 L4
  constraint midpoint L3 L5.start
  constraint coincident A7 L5.end
  constraint tangent A7 L5
  constraint midpoint L4 L6.start
  constraint coincident A7 L6.end
  constraint tangent A7 L6
  constraint coincident P0 L7.start
  constraint parallel L8 L9
  measures "d296" diameter of A4
  measures "d297" diameter of A5
  measures "d298" diameter of A7
  measures "d299" diameter of A8
  measures "d300" distance of P0 L9.end
extrude "Extrude43" add sketch "Sketch45" along normal blind 100 separate body contours A0 A2 A4 L4 L10 | A2 L0 A5 L4 L6 | A0 A2 L1 A4 A5 L2 L6 | A0 A2 A4 L10 | A2 A5 L4 L10 | A2 L0 A5 L4 | L1 A5 L6 | A0 A2 A4 L2 L5 | A0 A2 A4 L3 L10 | A2 A5 L7 L10 | A2 L3 L5 | L1 A5 A6 A8 L2 L6 | A2 L1 A5 L2 | A2 A5 L2 L5 | A2 L3 L10 | A5 L7 L8 L9 L10 | A2 A5 L3 L5 | A5 A6 A8 L2 L5 | A6 A7 A8 L5 L6 | A6 A7 A8 L2 L6 | A6 A7 A8 L2 L5 makes body 29
copy_body "Body->Comp15" bodies 28 removing the originals makes body 30 in component "old_component (13)"
copy_body "Body->Comp16" bodies 29 removing the originals makes body 31 in component "old_component (14)"
copy_body "CopyPasteBodies1" bodies 4 body 4 seen with x (0.267011, -0.094883, 0.959011) y (0.334841, 0.942275, 0) z (-0.903652, 0.321116, 0.283369) at (1606.6186, -543.6031, 946.8636) makes body 32 in component "Component2_1"
copy_body "CopyPasteBodies1'" bodies 5 body 5 seen with x (0.942275, -0.334841, 0) y (0.334841, 0.942275, 0) z (0, 0, 1) at (161.4797, -22.1078, -201.1799) makes body 33 in component "Component3_1"
copy_body "CopyPasteBodies1''" bodies 6 body 6 seen with x (1, 0, 0) y (0, 1, 0) z (0, 0, 1) at (161.4797, -22.1078, -136.1799) makes body 34 in component "base_link"
copy_body "CopyPasteBodies1'''" bodies 18 body 18 seen with x (0.34757, 0.936466, 0.047176) y (-0.250216, 0.141121, -0.95785) z (-0.903652, 0.321116, 0.283369) at (1381.7879, -413.7644, 792.7107) makes body 35 in component "Component5_1"
copy_body "CopyPasteBodies1''''" bodies 19 body 19 seen with x (0.34757, 0.936466, 0.047176) y (-0.741638, 0.305348, -0.597273) z (-0.573731, 0.172607, 0.800649) at (269.6365, 81.223, -924.0278) makes body 36 in component "Component6_1"
copy_body "CopyPasteBodies1'''''" bodies 20 body 20 seen with x (0.34757, 0.936466, 0.047176) y (-0.741638, 0.305348, -0.597273) z (-0.573731, 0.172607, 0.800649) at (327.5833, 63.7897, -1004.8934) makes body 37 in component "Component7_1"
copy_body "CopyPasteBodies1''''''" bodies 21 body 21 seen with x (0.71799, 0.576369, 0.390243) y (-0.394111, 0.798753, -0.454611) z (-0.573731, 0.172607, 0.800649) at (533.2687, 130.1276, -1120.3526) makes body 38 in component "Component8_1"
copy_body "CopyPasteBodies1'''''''" bodies 22 body 22 seen with x (0.71799, 0.576369, 0.390243) y (0.69493, -0.561735, -0.448916) z (-0.039528, 0.593509, -0.803856) at (-2006.1716, -2376.8812, 7254.5735) makes body 39 in component "Component9_1"
copy_body "CopyPasteBodies1''''''''" bodies 23 body 23 seen with x (-0.791305, 0.472641, 0.387875) y (0.610143, 0.651427, 0.450964) z (-0.039528, 0.593509, -0.803856) at (-2075.3249, -2103.5181, 7459.8054) makes body 40 in component "Component10_1"
copy_body "CopyPasteBodies1'''''''''" bodies 24 body 24 seen with x (0.66668, -0.729674, 0.152031) y (-0.610143, -0.651427, -0.450964) z (0.428094, 0.207888, -0.879499) at (-4981.8989, -279.6575, 7657.1742) makes body 41 in component "Component11_1"
copy_body "CopyPasteBodies1''''''''''" bodies 25 body 25 seen with x (0.413097, 0.224133, -0.882675) y (-0.610143, -0.651427, -0.450964) z (-0.676075, 0.724849, -0.13235) at (1312.0652, -3188.2376, 3343.111) makes body 42 in component "Component12_1"
copy_body "CopyPasteBodies1'''''''''''" bodies 26 body 26 seen with x (0.008638, 0.563686, -0.825944) y (-0.610143, -0.651427, -0.450964) z (-0.792245, 0.507839, 0.338302) at (1839.4358, -1946.8039, 836.3127) makes body 43 in component "Component13_1"
copy_body "CopyPasteBodies1''''''''''''" bodies 27 body 27 seen with x (0.351588, -0.732695, 0.582704) y (-0.610143, -0.651427, -0.450964) z (0.710008, -0.196979, -0.676083) at (-6490.517, 1910.2312, 6534.9519) makes body 44 in component "Component14_1"
copy_body "CopyPasteBodies1'''''''''''''" bodies 30 body 30 seen with x (0.999418, 0.01979, -0.027799) y (-0.019053, 0.999466, 0.026549) z (0.02831, -0.026004, 0.999261) at (-66.1814, 125.0503, -91.0962) makes body 45 in component "Component15_1"
copy_body "CopyPasteBodies1''''''''''''''" bodies 31 body 31 seen with x (0.999563, -0.016547, 0.024494) y (0.017101, 0.999599, -0.022558) z (-0.024111, 0.022967, 0.999445) at (55.8203, -107.4599, 79.7048) makes body 46 in component "Component16_1"
component "old_component (1)" placed x (0.267011, -0.094883, 0.959011) y (0.334841, 0.942275, 0) z (-0.903652, 0.321116, 0.283369) at (1606.6186, -543.6031, 946.8636)
component "old_component (2)" placed x (0.942275, -0.334841, 0) y (0.334841, 0.942275, 0) z (0, 0, 1) at (161.4797, -22.1078, -201.1799)
component "old_component" placed x (1, 0, 0) y (0, 1, 0) z (0, 0, 1) at (161.4797, -22.1078, -136.1799)
component "old_component (3)" placed x (0.34757, 0.936466, 0.047176) y (-0.250216, 0.141121, -0.95785) z (-0.903652, 0.321116, 0.283369) at (1381.7879, -413.7644, 792.7107)